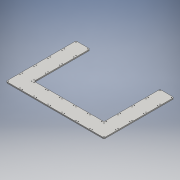
# Autodesk Inventor part: OuterFrame
Saved by Autodesk Inventor 2016 (Build 200138000, 138)
## iProperties
Created: 2016-05-22
Part Number: OuterFrame
Material: Generic
Document SubType Name: Modeling
Designer: Kurtis
Density: 1 g/cm^3
Appearance: Default
Author: Kurtis
Autodesk Inventor part; units mm, degrees
ref_plane "YZ Plane" through (0, 0, 0) normal (1, 0, 0) x (0, 1, 0)
ref_plane "XZ Plane" through (0, 0, 0) normal (0, 1, 0) x (-1, 0, 0)
ref_plane "XY Plane" through (0, 0, 0) normal (0, 0, 1) x (1, 0, 0)
sketch "Sketch1" plane through (0, 0, 0) normal (0, 0, 1) x (1, 0, 0)
  line L0 (0, 0) -> (420, 0)
  line L1 (420, 0) -> (420, 300)
  line L2 (420, 300) -> (360, 300)
  line L3 (360, 300) -> (360, 60)
  line L4 (360, 60) -> (60, 60)
  line L5 (60, 60) -> (60, 300)
  line L6 (60, 300) -> (0, 300)
  line L7 (0, 300) -> (0, 0)
  line L8 (0, 300) -> (0, 240) construction
  line L9 (0, 240) -> (0, 180) construction
  line L10 (0, 180) -> (0, 120) construction
  line L11 (0, 120) -> (0, 60) construction
  line L12 (420, 300) -> (420, 240) construction
  line L13 (420, 240) -> (420, 180) construction
  line L14 (420, 180) -> (420, 120) construction
  line L15 (420, 120) -> (420, 60) construction
  line L16 (60, 60) -> (120, 60) construction
  line L17 (120, 60) -> (180, 60) construction
  line L18 (180, 60) -> (240, 60) construction
  line L19 (240, 60) -> (300, 60) construction
  line L20 (300, 60) -> (360, 60) construction
  line L21 (0, 240) -> (60, 300) construction
  line L22 (0, 240) -> (60, 240) construction
  line L23 (0, 180) -> (60, 180) construction
  line L24 (0, 120) -> (60, 120) construction
  line L25 (0, 60) -> (60, 60) construction
  line L26 (60, 60) -> (60, 0) construction
  line L27 (0, 180) -> (60, 240) construction
  line L28 (0, 120) -> (60, 180) construction
  line L29 (0, 60) -> (60, 120) construction
  line L30 (0, 0) -> (60, 60) construction
  line L31 (120, 60) -> (120, 0) construction
  line L32 (180, 60) -> (180, 0) construction
  line L33 (240, 60) -> (240, 0) construction
  line L34 (300, 60) -> (300, 0) construction
  line L35 (360, 60) -> (360, 0) construction
  line L36 (360, 60) -> (420, 60) construction
  line L37 (360, 120) -> (420, 120) construction
  line L38 (420, 180) -> (360, 180) construction
  line L39 (420, 240) -> (360, 240) construction
  line L40 (60, 0) -> (120, 60) construction
  line L41 (120, 0) -> (180, 60) construction
  line L42 (180, 0) -> (240, 60) construction
  line L43 (240, 0) -> (300, 60) construction
  line L44 (300, 0) -> (360, 60) construction
  line L45 (360, 0) -> (420, 60) construction
  line L46 (360, 60) -> (420, 120) construction
  line L47 (360, 120) -> (420, 180) construction
  line L48 (360, 180) -> (420, 240) construction
  line L49 (360, 240) -> (420, 300) construction
  line L50 (5, 245) -> (55, 245) construction
  line L51 (55, 245) -> (55, 295) construction
  line L52 (55, 295) -> (5, 295) construction
  line L53 (5, 295) -> (5, 245) construction
  line L54 (5, 245) -> (55, 295) construction
  line L55 (55, 245) -> (5, 295) construction
  line L56 (5, 185) -> (55, 185) construction
  line L57 (55, 185) -> (55, 235) construction
  line L58 (55, 235) -> (5, 235) construction
  line L59 (5, 235) -> (5, 185) construction
  line L60 (5, 185) -> (55, 235) construction
  line L61 (55, 185) -> (5, 235) construction
  line L62 (5, 125) -> (55, 125) construction
  line L63 (55, 125) -> (55, 175) construction
  line L64 (55, 175) -> (5, 175) construction
  line L65 (5, 175) -> (5, 125) construction
  line L66 (5, 125) -> (55, 175) construction
  line L67 (55, 125) -> (5, 175) construction
  line L68 (5, 65) -> (55, 65) construction
  line L69 (55, 65) -> (55, 115) construction
  line L70 (55, 115) -> (5, 115) construction
  line L71 (5, 115) -> (5, 65) construction
  line L72 (5, 65) -> (55, 115) construction
  line L73 (55, 65) -> (5, 115) construction
  line L74 (5, 5) -> (55, 5) construction
  line L75 (55, 5) -> (55, 55) construction
  line L76 (55, 55) -> (5, 55) construction
  line L77 (5, 55) -> (5, 5) construction
  line L78 (5, 5) -> (55, 55) construction
  line L79 (55, 5) -> (5, 55) construction
  line L80 (65, 5) -> (115, 5) construction
  line L81 (115, 5) -> (115, 55) construction
  line L82 (115, 55) -> (65, 55) construction
  line L83 (65, 55) -> (65, 5) construction
  line L84 (65, 5) -> (115, 55) construction
  line L85 (115, 5) -> (65, 55) construction
  line L86 (125, 5) -> (175, 5) construction
  line L87 (175, 5) -> (175, 55) construction
  line L88 (175, 55) -> (125, 55) construction
  line L89 (125, 55) -> (125, 5) construction
  line L90 (125, 5) -> (175, 55) construction
  line L91 (175, 5) -> (125, 55) construction
  line L92 (185, 5) -> (235, 5) construction
  line L93 (235, 5) -> (235, 55) construction
  line L94 (235, 55) -> (185, 55) construction
  line L95 (185, 55) -> (185, 5) construction
  line L96 (185, 5) -> (235, 55) construction
  line L97 (235, 5) -> (185, 55) construction
  line L98 (245, 5) -> (295, 5) construction
  line L99 (295, 5) -> (295, 55) construction
  line L100 (295, 55) -> (245, 55) construction
  line L101 (245, 55) -> (245, 5) construction
  line L102 (245, 5) -> (295, 55) construction
  line L103 (295, 5) -> (245, 55) construction
  line L104 (305, 5) -> (355, 5) construction
  line L105 (355, 5) -> (355, 55) construction
  line L106 (355, 55) -> (305, 55) construction
  line L107 (305, 55) -> (305, 5) construction
  line L108 (305, 5) -> (355, 55) construction
  line L109 (355, 5) -> (305, 55) construction
  line L110 (365, 5) -> (415, 5) construction
  line L111 (415, 5) -> (415, 55) construction
  line L112 (415, 55) -> (365, 55) construction
  line L113 (365, 55) -> (365, 5) construction
  line L114 (365, 5) -> (415, 55) construction
  line L115 (415, 5) -> (365, 55) construction
  line L116 (365, 65) -> (415, 65) construction
  line L117 (415, 65) -> (415, 115) construction
  line L118 (415, 115) -> (365, 115) construction
  line L119 (365, 115) -> (365, 65) construction
  line L120 (365, 65) -> (415, 115) construction
  line L121 (415, 65) -> (365, 115) construction
  line L122 (365, 125) -> (415, 125) construction
  line L123 (415, 125) -> (415, 175) construction
  line L124 (415, 175) -> (365, 175) construction
  line L125 (365, 175) -> (365, 125) construction
  line L126 (365, 125) -> (415, 175) construction
  line L127 (415, 125) -> (365, 175) construction
  line L128 (365, 185) -> (415, 185) construction
  line L129 (415, 185) -> (415, 235) construction
  line L130 (415, 235) -> (365, 235) construction
  line L131 (365, 235) -> (365, 185) construction
  line L132 (365, 185) -> (415, 235) construction
  line L133 (415, 185) -> (365, 235) construction
  line L134 (365, 245) -> (415, 245) construction
  line L135 (415, 245) -> (415, 295) construction
  line L136 (415, 295) -> (365, 295) construction
  line L137 (365, 295) -> (365, 245) construction
  line L138 (365, 245) -> (415, 295) construction
  line L139 (415, 245) -> (365, 295) construction
  circle A0 centre (5, 295) radius 1.5
  circle A1 centre (55, 295) radius 1.5
  circle A2 centre (55, 245) radius 1.5
  circle A3 centre (5, 245) radius 1.5
  circle A4 centre (5, 5) radius 1.5
  circle A5 centre (55, 5) radius 1.5
  circle A6 centre (5, 55) radius 1.5
  circle A7 centre (55, 55) radius 1.5
  circle A8 centre (235, 55) radius 1.5
  circle A9 centre (185, 55) radius 1.5
  circle A10 centre (185, 5) radius 1.5
  circle A11 centre (235, 5) radius 1.5
  circle A12 centre (365, 55) radius 1.5
  circle A13 centre (415, 55) radius 1.5
  circle A14 centre (415, 5) radius 1.5
  circle A15 centre (365, 5) radius 1.5
  circle A16 centre (365, 295) radius 1.5
  circle A17 centre (415, 295) radius 1.5
  circle A18 centre (365, 245) radius 1.5
  circle A19 centre (415, 245) radius 1.5
  circle A20 centre (365, 235) radius 1.5
  circle A21 centre (415, 235) radius 1.5
  circle A22 centre (365, 185) radius 1.5
  circle A23 centre (415, 185) radius 1.5
  circle A24 centre (365, 175) radius 1.5
  circle A25 centre (415, 175) radius 1.5
  circle A26 centre (365, 125) radius 1.5
  circle A27 centre (415, 125) radius 1.5
  circle A28 centre (365, 115) radius 1.5
  circle A29 centre (415, 115) radius 1.5
  circle A30 centre (365, 65) radius 1.5
  circle A31 centre (415, 65) radius 1.5
  circle A32 centre (305, 55) radius 1.5
  circle A33 centre (355, 55) radius 1.5
  circle A34 centre (305, 5) radius 1.5
  circle A35 centre (355, 5) radius 1.5
  circle A36 centre (295, 55) radius 1.5
  circle A37 centre (245, 55) radius 1.5
  circle A38 centre (245, 5) radius 1.5
  circle A39 centre (295, 5) radius 1.5
  circle A40 centre (175, 55) radius 1.5
  circle A41 centre (125, 55) radius 1.5
  circle A42 centre (125, 5) radius 1.5
  circle A43 centre (175, 5) radius 1.5
  circle A44 centre (115, 55) radius 1.5
  circle A45 centre (65, 55) radius 1.5
  circle A46 centre (65, 5) radius 1.5
  circle A47 centre (115, 5) radius 1.5
  circle A48 centre (5, 65) radius 1.5
  circle A49 centre (55, 65) radius 1.5
  circle A50 centre (55, 115) radius 1.5
  circle A51 centre (5, 115) radius 1.5
  circle A52 centre (5, 125) radius 1.5
  circle A53 centre (55, 125) radius 1.5
  circle A54 centre (5, 175) radius 1.5
  circle A55 centre (55, 175) radius 1.5
  circle A56 centre (5, 185) radius 1.5
  circle A57 centre (55, 185) radius 1.5
  circle A58 centre (5, 235) radius 1.5
  circle A59 centre (55, 235) radius 1.5
  point P0 (30, 270)
  point P1 (30, 210)
  point P2 (30, 150)
  point P3 (30, 90)
  point P4 (30, 30)
  point P5 (90, 30)
  point P6 (150, 30)
  point P7 (210, 30)
  point P8 (270, 30)
  point P9 (330, 30)
  point P10 (390, 30)
  point P11 (390, 90)
  point P12 (390, 150)
  point P13 (390, 210)
  point P14 (390, 270)
  dimension "d0" = 420
  dimension "d1" = 300
  dimension "d2" = 60
  dimension "d3" = 240
  dimension "d4" = 300
  dimension "d5" = 240
  dimension "d6" = 60
  dimension "d7" = 60
  dimension "d8" = 60
  dimension "d9" = 60
  dimension "d10" = 60
  dimension "d11" = 60
  dimension "d12" = 60
  dimension "d13" = 60
  dimension "d14" = 60
  dimension "d15" = 60
  dimension "d16" = 60
  dimension "d17" = 60
  dimension "d20" = 50
  dimension "d21" = 50
  dimension "d22" = 50
  dimension "d23" = 50
  dimension "d24" = 50
  dimension "d25" = 50
  dimension "d26" = 50
  dimension "d27" = 50
  dimension "d28" = 50
  dimension "d29" = 50
  dimension "d30" = 50
  dimension "d31" = 50
  dimension "d32" = 50
  dimension "d33" = 50
  dimension "d34" = 50
  dimension "d35" = 50
  dimension "d36" = 50
  dimension "d37" = 50
  dimension "d38" = 50
  dimension "d39" = 50
  dimension "d40" = 50
  dimension "d41" = 50
  dimension "d42" = 50
  dimension "d43" = 50
  dimension "d44" = 50
  dimension "d45" = 50
  dimension "d46" = 50
  dimension "d47" = 50
  dimension "d48" = 50
  dimension "d49" = 50
  dimension "d50" = 3
  dimension "d51" = 3
  dimension "d52" = 3
  dimension "d53" = 3
  dimension "d54" = 3
  dimension "d55" = 3
  dimension "d56" = 3
  dimension "d57" = 3
  dimension "d58" = 3
  dimension "d59" = 3
  dimension "d60" = 3
  dimension "d61" = 3
  dimension "d62" = 3
  dimension "d63" = 3
  dimension "d64" = 3
  dimension "d65" = 3
  constraints: 280 end point, 60 centre point, 59 coincident, 47 midpoint, 32 equal length, 29 perpendicular, 29 point on line, 17 horizontal
  measures "d0" distance of L0.start L0.end
  measures "d1" distance of L0.end L1.end
  measures "d2" distance of L1.end L2.end
  measures "d3" distance of L2.end L3.end
  measures "d4" distance of L3.end L4.end
  measures "d5" distance of L4.end L5.end
  measures "d6" distance of L6.end L8.end
  measures "d7" distance of L8.end L9.end
  measures "d8" distance of L9.end L10.end
  measures "d9" distance of L10.end L11.end
  measures "d10" distance of L1.end L12.end
  measures "d11" distance of L12.end L13.end
  measures "d12" distance of L13.end L14.end
  measures "d13" distance of L14.end L15.end
  measures "d14" distance of L4.end L16.end
  measures "d15" distance of L16.end L17.end
  measures "d16" distance of L17.end L18.end
  measures "d17" distance of L18.end L19.end
  measures "d20" distance of L52.end L51.end
  measures "d21" distance of L51.end L50.end
  measures "d22" distance of L58.end L57.end
  measures "d23" distance of L57.end L56.end
  measures "d24" distance of L64.end L63.end
  measures "d25" distance of L63.end L62.end
  measures "d26" distance of L70.end L69.end
  measures "d27" distance of L69.end L68.end
  measures "d28" distance of L76.end L75.end
  measures "d29" distance of L75.end L74.end
  measures "d30" distance of L82.end L81.end
  measures "d31" distance of L81.end L80.end
  measures "d32" distance of L88.end L87.end
  measures "d33" distance of L87.end L86.end
  measures "d34" distance of L94.end L93.end
  measures "d35" distance of L93.end L92.end
  measures "d36" distance of L100.end L99.end
  measures "d37" distance of L99.end L98.end
  measures "d38" distance of L106.end L105.end
  measures "d39" distance of L105.end L104.end
  measures "d40" distance of L112.end L111.end
  measures "d41" distance of L111.end L110.end
  measures "d42" distance of L118.end L117.end
  measures "d43" distance of L117.end L116.end
  measures "d44" distance of L124.end L123.end
  measures "d45" distance of L123.end L122.end
  measures "d46" distance of L130.end L129.end
  measures "d47" distance of L129.end L128.end
  measures "d48" distance of L136.end L135.end
  measures "d49" distance of L135.end L134.end
  measures "d50" diameter of A0
  measures "d51" diameter of A1
  measures "d52" diameter of A2
  measures "d53" diameter of A3
  measures "d54" diameter of A4
  measures "d55" diameter of A5
  measures "d56" diameter of A6
  measures "d57" diameter of A7
  measures "d58" diameter of A8
  measures "d59" diameter of A9
  measures "d60" diameter of A10
  measures "d61" diameter of A11
  measures "d62" diameter of A12
  measures "d63" diameter of A13
  measures "d64" diameter of A14
  measures "d65" diameter of A15
extrude "Frame" add sketch "Sketch1" along normal blind 5
fillet "Fillet1" radius 5 8 edges at (60, 60, 2.5) (360, 60, 2.5) (420, 0, 2.5) (360, 300, 2.5) (420, 300, 2.5) (0, 0, 2.5) (0, 300, 2.5) (60, 300, 2.5)
body "Solid2"
